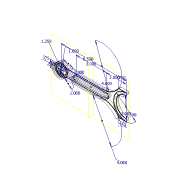
# Autodesk Inventor part: Part1
Saved by Autodesk Inventor 2017 (Build 210142000, 142)
## iProperties
Created: 2018-11-02
Part Number: Part1
Material: Generic
Document SubType Name: Modeling
Designer: jpb34
Density: 1 g/cm^3
Appearance: Default
Author: jpb34
Autodesk Inventor part; units mm, degrees
sketch "Sketch1" plane through (0, 0, 0) normal (0, 0, 1) x (1, 0, 0)
  circle A0 centre (-76.2, 0) radius 15.875
  line L0 (-38.1, 0) -> (38.1, 0) construction
  line L1 (-38.1, -6.35) -> (38.1, -6.35)
  line L2 (38.1, 6.35) -> (-38.1, 6.35)
  arc A1 (-38.1, 6.35) -> (-38.1, -6.35) centre (-38.1, 0) ccw
  arc A2 (38.1, -6.35) -> (38.1, 6.35) centre (38.1, 0) ccw
  arc A3 (88.9, 31.75) -> (88.9, -31.75) centre (88.9, 0) ccw
  circle A4 centre (-76.2, 0) radius 12.7
  arc A5 (88.9, 25.4) -> (88.9, -25.4) centre (88.9, 0) ccw
  line L3 (88.9, 31.75) -> (88.9, 25.4)
  line L4 (88.9, -25.4) -> (88.9, -31.75)
  line L5 (88.9, 31.75) -> (69.85, 31.75)
  line L6 (88.9, -31.75) -> (69.85, -31.75)
  line L7 (-58.2395, 9.525) -> (27.8487, 9.525)
  line L8 (-59.2632, -9.525) -> (27.8487, -9.525)
  arc A6 (27.8487, 9.525) -> (69.85, 31.75) centre (27.8487, 60.325) ccw
  arc A7 (69.85, -31.75) -> (27.8487, -9.525) centre (27.8487, -60.325) ccw
  arc A8 (-66.2219, 12.3472) -> (-58.2395, 9.525) centre (-58.2395, 22.225) ccw
  arc A9 (-57.1021, -9.525) -> (-66.1904, -12.3216) centre (-58.1827, -22.1789) ccw
  point P0 (0, 0)
  point P1 (0, 0)
  dimension "d0" = 31.75
  dimension "d1" = 25.4
  dimension "d2" = 12.7
  dimension "d3" = 76.2
  dimension "d4" = 165.1
  dimension "d5" = 50.8
  dimension "d6" = 63.5
  dimension "d7" = 50.8
  dimension "d8" = 19.05
  dimension "d9" = 19.05
  dimension "d12" = 19.05
  dimension "d13" = 9.525
  dimension "d15" = 101.6
  dimension "d16" = 101.6
  dimension "d17" = 25.4
  dimension "d18" = 25.4
  dimension "d19" = 0
  constraints: 20 end point, 19 point on circle, 11 tangent, 10 centre point, 4 horizontal, 3 coincident, 2 parallel, 2 vertical, 1 midpoint, 1 point on line
  measures "d0" diameter of A0
  measures "d1" diameter of A4
  measures "d2" distance between parallel lines of L2 L1
  measures "d3" distance of L2.start L2.end
  measures "d4" distance of A3.centre A0.centre
  measures "d5" horizontal distance of A3.centre L2.start
  measures "d6" diameter of A3
  measures "d7" diameter of A5
  measures "d8" distance of L3.start L5.end
  measures "d9" distance of L4.end L6.end
  measures "d12" distance between parallel lines of L8 L7
  measures "d13" distance from line of L7 point (0, 0)
  measures "d15" diameter of A6
  measures "d16" diameter of A7
  measures "d17" diameter of A9
  measures "d18" diameter of A8
  measures "d19" vertical distance of A0.centre point (0, 0)
extrude "Base" add sketch "Sketch1" along normal mid plane 12.7 contours A0 | A0 A8 L7 A6 L5 A3 L6 A7 L8 A9 | L3 A5 L4 A3
extrude "Extrusion2" add sketch "Sketch1" along normal mid plane 6.35 contours A1 L2 A2 L1
sketch "Sketch2" plane through (0, 0, 0) normal (0, 0, 1) x (1, 0, 0)
  arc A0 (-38.1, 6.35) -> (-38.1, -6.35) centre (-38.1, 0) ccw projected
  line L0 (-38.1, 6.35) -> (38.1, 6.35) projected
  arc A1 (38.1, -6.35) -> (38.1, 6.35) centre (38.1, 0) ccw projected
  line L1 (38.1, -6.35) -> (-38.1, -6.35) projected
  circle A2 centre (-76.2, 0) radius 12.7 projected
  line L2 (88.9, -31.75) -> (88.9, -25.4) projected
  arc A3 (88.9, 25.4) -> (88.9, -25.4) centre (88.9, 0) ccw projected
  line L3 (88.9, 25.4) -> (88.9, 31.75) projected
  line L4 (88.9, 31.75) -> (69.85, 31.75) projected
  arc A4 (27.8487, 9.525) -> (69.85, 31.75) centre (27.8487, 60.325) ccw projected
  line L5 (27.8487, 9.525) -> (-58.2395, 9.525) projected
  arc A5 (-66.2219, 12.3472) -> (-58.2395, 9.525) centre (-58.2395, 22.225) ccw projected
  arc A6 (-66.2219, 12.3472) -> (-66.1904, -12.3216) centre (-76.2, 0) ccw projected
  arc A7 (-57.1021, -9.525) -> (-66.1904, -12.3216) centre (-58.1827, -22.1789) ccw projected
  line L6 (-57.1021, -9.525) -> (27.8487, -9.525) projected
  arc A8 (69.85, -31.75) -> (27.8487, -9.525) centre (27.8487, -60.325) ccw projected
  line L7 (69.85, -31.75) -> (88.9, -31.75) projected
  arc A9 (-38.1, 6.35) -> (-38.1, -6.35) centre (-38.1, 0) ccw projected
  line L8 (-38.1, 6.35) -> (38.1, 6.35) projected
  arc A10 (38.1, -6.35) -> (38.1, 6.35) centre (38.1, 0) ccw projected
  line L9 (38.1, -6.35) -> (-38.1, -6.35) projected
  circle A11 centre (-76.2, 0) radius 12.7 projected
  line L10 (88.9, -31.75) -> (88.9, -25.4) projected
  arc A12 (88.9, 25.4) -> (88.9, -25.4) centre (88.9, 0) ccw projected
  line L11 (88.9, 25.4) -> (88.9, 31.75) projected
  line L12 (88.9, 31.75) -> (69.85, 31.75) projected
  arc A13 (27.8487, 9.525) -> (69.85, 31.75) centre (27.8487, 60.325) ccw projected
  line L13 (27.8487, 9.525) -> (-58.2395, 9.525) projected
  arc A14 (-66.2219, 12.3472) -> (-58.2395, 9.525) centre (-58.2395, 22.225) ccw projected
  arc A15 (-66.2219, 12.3472) -> (-66.1904, -12.3216) centre (-76.2, 0) ccw projected
  arc A16 (-57.1021, -9.525) -> (-66.1904, -12.3216) centre (-58.1827, -22.1789) ccw projected
  line L14 (-57.1021, -9.525) -> (27.8487, -9.525) projected
  arc A17 (69.85, -31.75) -> (27.8487, -9.525) centre (27.8487, -60.325) ccw projected
  line L15 (69.85, -31.75) -> (88.9, -31.75) projected
  circle A18 centre (-76.2, 0) radius 12.7
  circle A19 centre (-76.2, 0) radius 15.875
  circle A20 centre (-76.2, 0) radius 15.875
  point P0 (0, 0)
  constraints: 3 centre point, 3 coincident, 1 concentric
body "Solid1"
